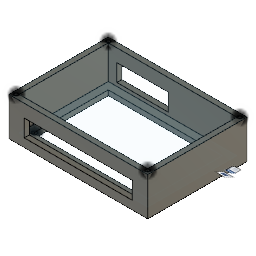
relaybox2 (1) (Autodesk Fusion 360 design; units mm, degrees)
part number: 2025-12-15-16-26-34-324
Autodesk Fusion 360 part; units mm, degrees
sketch "Sketch1" plane through (0, 0, 0) normal (0, 0, 1) x (1, 0, 0)
  line L0 (40.5, 29) -> (-40.5, 29)
  line L1 (-40.5, 29) -> (-40.5, -29)
  line L2 (-40.5, -29) -> (40.5, -29)
  line L3 (40.5, -29) -> (40.5, 29)
  line L4 (40.5, 29) -> (-40.5, -29) construction
  line L5 (-40.5, 29) -> (40.5, -29) construction
  dimension "d1" = 81
  dimension "d2" = 58
  constraint horizontal L0
  constraint perpendicular L0 L1
  constraint parallel L0 L2
  constraint parallel L1 L3
  constraint coincident L4 origin
  constraint coincident L5 origin
  measures "d1" distance of L1.end L2.end
  measures "d2" distance of L0.end L1.end
extrude "Extrude1" add sketch "Sketch1" along normal blind 22.5
sketch "Sketch2" plane through (0, 0, 22.5) normal (0, 0, 1) x (-1, 0, 0)
  line L0 (-40.5, 29) -> (-40.5, -29)
  line L1 (-40.5, -29) -> (40.5, -29)
  line L2 (40.5, -29) -> (40.5, 29)
  line L3 (40.5, 29) -> (-40.5, 29)
  line L4 (-37.5, -26) -> (37.5, -26)
  line L5 (37.5, -26) -> (37.5, 26)
  line L6 (37.5, 26) -> (-37.5, 26)
  line L7 (-37.5, 26) -> (-37.5, -26)
  line L8 (-37.5, -26) -> (37.5, 26) construction
  line L9 (37.5, -26) -> (-37.5, 26) construction
  dimension "d5" = 75
  dimension "d6" = 52
  constraint horizontal L4
  constraint perpendicular L4 L5
  constraint parallel L4 L6
  constraint parallel L5 L7
  constraint coincident L8 origin
  constraint coincident L9 origin
  measures "d5" distance of L5.end L6.end
  measures "d6" distance of L4.end L5.end
extrude "Extrude2" cut sketch "Sketch2" against normal blind 19.5 contours L4 L5 L6 L7
sketch "Sketch3" plane through (0, 0, 0) normal (0, 0, -1) x (1, 0, 0)
  line L0 (40.5, -29) -> (40.5, 29)
  line L1 (40.5, 29) -> (-40.5, 29)
  line L2 (-40.5, 29) -> (-40.5, -29)
  line L3 (-40.5, -29) -> (40.5, -29)
  line L4 (33.25, 21.75) -> (-33.25, 21.75)
  line L5 (-33.25, 21.75) -> (-33.25, -21.75)
  line L6 (-33.25, -21.75) -> (33.25, -21.75)
  line L7 (33.25, -21.75) -> (33.25, 21.75)
  line L8 (33.25, 21.75) -> (-33.25, -21.75) construction
  line L9 (-33.25, 21.75) -> (33.25, -21.75) construction
  dimension "d9" = 66.5
  dimension "d10" = 43.5
  constraint horizontal L4
  constraint perpendicular L4 L5
  constraint parallel L4 L6
  constraint parallel L5 L7
  constraint coincident L8 origin
  constraint coincident L9 origin
  measures "d9" distance of L5.end L6.end
  measures "d10" distance of L4.end L5.end
sketch "Sketch4" plane through (0, 0, 0) normal (0, 0, -1) x (1, 0, 0)
extrude "Extrude3" cut sketch "Sketch3" against normal blind 3 contours L4 L5 L6 L7
sketch "Sketch5" plane through (0, 0, 3) normal (0, 0, 1) x (-1, 0, 0)
  line L0 (-33.25, 21.75) -> (33.25, 21.75)
  line L1 (33.25, 21.75) -> (33.25, -21.75)
  line L2 (33.25, -21.75) -> (-33.25, -21.75)
  line L3 (-33.25, -21.75) -> (-33.25, 21.75)
  line L4 (-37.5, 26) -> (-37.5, -26)
  line L5 (-37.5, -26) -> (37.5, -26)
  line L6 (37.5, -26) -> (37.5, 26)
  line L7 (37.5, 26) -> (-37.5, 26)
  circle A0 centre (35.875, -24.375) radius 1.5
  dimension "d13" = 3
  dimension "d14" = 1.625
  dimension "d15" = 1.625
  measures "d13" diameter of A0
  measures "d14" distance of L5 A0.centre
  measures "d15" distance of L6 A0.centre
sketch "Sketch6" plane through (0, 0, 3) normal (0, 0, 1) x (-1, 0, 0)
  circle A0 centre (-35.875, -24.375) radius 1.5
  line L0 (-37.5, -26) -> (37.5, -26)
  line L1 (-37.5, 26) -> (-37.5, -26)
  circle A1 centre (-35.875, 24.375) radius 1.5
  line L2 (37.5, 26) -> (-37.5, 26)
  circle A2 centre (35.875, 24.375) radius 1.5
  line L3 (37.5, -26) -> (37.5, 26)
  dimension "d16" = 3
  dimension "d17" = 1.625
  dimension "d18" = 1.625
  dimension "d19" = 3
  dimension "d20" = 1.625
  dimension "d21" = 1.625
  dimension "d25" = 3
  dimension "d26" = 1.625
  dimension "d27" = 1.625
  measures "d16" diameter of A0
  measures "d17" distance of A0.centre L0
  measures "d18" distance of A0.centre L1
  measures "d19" diameter of A1
  measures "d20" distance of L1 A1.centre
  measures "d21" distance of A1.centre L2
  measures "d25" diameter of A2
  measures "d26" distance of L2 A2.centre
  measures "d27" distance of A2.centre L3
sketch "Sketch8" plane through (0, -29, 0) normal (0, -1, 0) x (1, 0, 0)
  line L0 (-40.5, 0) -> (40.5, 0)
  line L1 (40.5, 0) -> (40.5, 22.5)
  line L2 (40.5, 22.5) -> (-40.5, 22.5)
  line L3 (-40.5, 22.5) -> (-40.5, 0)
  line L4 (31.5, 15) -> (-31.5, 15)
  line L5 (-31.5, 15) -> (-31.5, 5)
  line L6 (-31.5, 5) -> (31.5, 5)
  line L7 (31.5, 5) -> (31.5, 15)
  line L8 (31.5, 15) -> (-31.5, 5) construction
  line L9 (-31.5, 15) -> (31.5, 5) construction
  point P0 (0, 10)
  dimension "d30" = 63
  dimension "d31" = 10
  dimension "d33" = 15
  constraint horizontal L4
  constraint perpendicular L4 L5
  constraint parallel L4 L6
  constraint parallel L5 L7
  constraint coincident L8 P0
  constraint coincident L9 P0
  measures "d30" distance of L5.end L6.end
  measures "d31" distance of L4.end L5.end
  measures "d33" distance of L0 L4
extrude "Extrude5" cut sketch "Sketch8" against normal blind 3 contours L4 L5 L6 L7
sketch "Sketch9" plane through (0, 29, 0) normal (0, 1, 0) x (-1, 0, 0)
  line L0 (-40.5, 0) -> (40.5, 0)
  line L1 (40.5, 0) -> (40.5, 22.5)
  line L2 (40.5, 22.5) -> (-40.5, 22.5)
  line L3 (-40.5, 22.5) -> (-40.5, 0)
  line L4 (32.5, 15) -> (2.5, 15)
  line L5 (2.5, 15) -> (2.5, 5)
  line L6 (2.5, 5) -> (32.5, 5)
  line L7 (32.5, 5) -> (32.5, 15)
  line L8 (32.5, 15) -> (2.5, 5) construction
  line L9 (2.5, 15) -> (32.5, 5) construction
  point P0 (17.5, 10)
  dimension "d36" = 30
  dimension "d37" = 10
  dimension "d38" = 8
  dimension "d39" = 15
  constraint horizontal L4
  constraint perpendicular L4 L5
  constraint parallel L4 L6
  constraint parallel L5 L7
  constraint coincident L8 P0
  constraint coincident L9 P0
  measures "d36" distance of L5.end L6.end
  measures "d37" distance of L4.end L5.end
  measures "d38" distance of L1 L7
  measures "d39" distance of L0 L4
extrude "Extrude6" cut sketch "Sketch9" against normal blind 3 contours L4 L5 L6 L7
sketch "Sketch11" plane through (0, 0, 22.5) normal (0, 0, 1) x (-1, 0, 0)
  line L0 (37.5, -26) -> (-37.5, -26)
  line L1 (-37.5, -26) -> (-37.5, 26)
  line L2 (-37.5, 26) -> (37.5, 26)
  line L3 (37.5, 26) -> (37.5, -26)
  line L4 (-40.5, 29) -> (-40.5, -29)
  line L5 (-40.5, -29) -> (40.5, -29)
  line L6 (40.5, -29) -> (40.5, 29)
  line L7 (40.5, 29) -> (-40.5, 29)
  circle A0 centre (38.375, -26.875) radius 1
  circle A1 centre (38.375, 26.875) radius 1
  circle A2 centre (-38.375, 26.875) radius 1
  circle A3 centre (-38.375, -26.875) radius 1
  dimension "d56" = 2
  dimension "d57" = 2
  dimension "d58" = 2
  dimension "d59" = 2
  dimension "d60" = 2.125
  dimension "d61" = 2.125
  dimension "d62" = 2.125
  dimension "d63" = 2.125
  dimension "d64" = 2.125
  dimension "d65" = 2.125
  dimension "d66" = 2.125
  dimension "d67" = 2.125
  measures "d56" diameter of A0
  measures "d57" diameter of A1
  measures "d58" diameter of A2
  measures "d59" diameter of A3
  measures "d60" distance of L5 A0.centre
  measures "d61" distance of L6 A0.centre
  measures "d62" distance of L5 A3.centre
  measures "d63" distance of L4 A3.centre
  measures "d64" distance of L4 A2.centre
  measures "d65" distance of L7 A2.centre
  measures "d66" distance of L7 A1.centre
  measures "d67" distance of L6 A1.centre
hole "Hole1" at (-38.375, 26.875, 22.5) at (38.375, 26.875, 22.5) at (38.375, -26.875, 22.5) at (-38.375, -26.875, 22.5) direction (0, 0, -1) diameter 1.6256 depth 5 tip angle 180
thread "Thread1" "ISO Metric profile 2.0 M2x0.4 M2x0.4 6H" thread offset 0 thread depth 5.9436
sketch "Sketch12" plane through (0, 0, 0) normal (0, 0, 1) x (1, 0, 0)
sketch "Sketch13" plane through (0, 0, 3) normal (0, 0, 1) x (-1, 0, 0)
  line L0 (-33.25, 21.75) -> (33.25, 21.75)
  line L1 (33.25, 21.75) -> (33.25, -21.75)
  line L2 (33.25, -21.75) -> (-33.25, -21.75)
  line L3 (-33.25, -21.75) -> (-33.25, 21.75)
  line L4 (-37.5, 26) -> (-37.5, -26)
  line L5 (-37.5, -26) -> (37.5, -26)
  line L6 (37.5, -26) -> (37.5, 26)
  line L7 (37.5, 26) -> (-37.5, 26)
  circle A0 centre (33, 21.5) radius 1.25
  dimension "d73" = 2.5
  dimension "d74" = 4.5
  dimension "d75" = 4.5
  measures "d73" diameter of A0
  measures "d74" distance of L7 A0.centre
  measures "d75" distance of L6 A0.centre
sketch "Sketch14" plane through (0, 0, 3) normal (0, 0, 1) x (-1, 0, 0)
